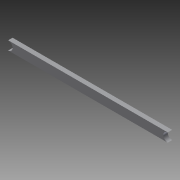
# Autodesk Inventor part: bar
Saved by Autodesk Inventor 2011 (Build 150239000, 239)
## iProperties
Created: 2011-07-10
Part Number: bar
Document SubType Name: Modeling
Designer: adowning
Density: 1 g/cm^3
Author: adowning
Autodesk Inventor part; units mm, degrees
ref_plane "YZ Plane" through (0, 0, 0) normal (1, 0, 0) x (0, 1, 0)
ref_plane "XZ Plane" through (0, 0, 0) normal (0, 1, 0) x (-1, 0, 0)
ref_plane "XY Plane" through (0, 0, 0) normal (0, 0, 1) x (1, 0, 0)
sketch "Sketch1" plane through (0, 0, 0) normal (0, 0, 1) x (1, 0, 0)
  line L0 (-39.1771, 0) -> (75.1229, 0)
  line L1 (75.1229, 0) -> (75.1229, -6.35)
  line L2 (75.1229, -6.35) -> (-39.1771, -6.35)
  line L3 (-39.1771, -6.35) -> (-39.1771, 0)
  point P0 (0, 0)
  dimension "d0" = 114.3
  dimension "d1" = 6.35
  constraints: 8 end point, 2 parallel, 1 horizontal, 1 perpendicular
  measures "d0" distance of L1.end L2.end
  measures "d1" distance of L0.end L1.end
extrude "Extrusion1" add sketch "Sketch1" along normal blind 6.35
sketch "Sketch2" plane through (0, 0, 6.35) normal (0, 0, 1) x (1, 0, 0)
  line L0 (75.1229, 0) -> (75.1229, -6.35) projected
  line L1 (-39.1771, -6.35) -> (-39.1771, 0) projected
  line L2 (-39.1771, 0) -> (-39.1771, -3.175)
  line L3 (-39.1771, -3.175) -> (75.1229, -3.175)
  circle A0 centre (-39.1771, -3.175) radius 3.175
  circle A1 centre (75.1229, -3.175) radius 3.175
  point P0 (0, 0)
  dimension "d4" = 3.175
  constraints: 4 end point, 2 coincident, 2 midpoint, 2 vertical alignment, 4 other
  measures "d4" distance of L1.end L2.end
extrude "Extrusion2" cut sketch "Sketch2" against normal blind 6.35
sketch "Sketch3" plane through (0, 0, 6.35) normal (0, 0, 1) x (1, 0, 0)
  arc A0 (-39.1771, -6.35) -> (-39.1771, 0) centre (-39.1771, -3.175) ccw projected
  line L0 (75.1229, -6.35) -> (-39.1771, -6.35) projected
  arc A1 (75.1229, 0) -> (75.1229, -6.35) centre (75.1229, -3.175) ccw projected
  line L1 (-39.1771, 0) -> (75.1229, 0) projected
  point P0 (0, 0)
extrude "Extrusion3" cut sketch "Sketch3" against normal blind 3.175
body "Solid1"
